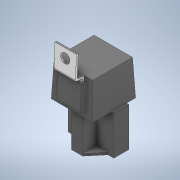
# Autodesk Inventor part: gooacc_30A_spdt
Saved by Autodesk Inventor 2020.2 (Build 242310000, 310)
## iProperties
Created: 2020-04-10
Part Number: gooacc_30A_spdt
Material: PC/ABS Plastic
Document SubType Name: Modeling
Designer: agmlego
Mass: 12.6544 g
Surface Area: 87.4119 cm^2
Volume: 35.4195 cm^3
Density: 0.357273 g/cm^3
Appearance: Smooth - Black
Author: agmlego
Autodesk Inventor part; units mm, degrees
ref_plane "YZ Plane" through (0, 0, 0) normal (1, 0, 0) x (0, 1, 0)
ref_plane "XZ Plane" through (0, 0, 0) normal (0, 1, 0) x (-1, 0, 0)
ref_plane "XY Plane" through (0, 0, 0) normal (0, 0, 1) x (1, 0, 0)
sketch "Sketch1" plane through (0, 0, 0) normal (0, 1, 0) x (-1, 0, 0)
  line L0 (0, 0) -> (27.2, 0)
  line L1 (27.2, 0) -> (27.2, -28.2)
  line L2 (27.2, -28.2) -> (0, -28.2)
  line L3 (0, -28.2) -> (0, 0)
  dimension "d0" = 27.2
  dimension "d1" = 28.2
  constraints: 8 end point, 2 parallel, 1 horizontal, 1 perpendicular
  measures "d0" distance of L0.start L0.end
  measures "d1" distance of L2.end L0.start
extrude "Extrusion1" add sketch "Sketch1" along normal blind 24.9
draft "FaceDraft1" angle 2.5 pull direction (0, 1, 0) faces at (-18.1333, 8.3, 0) (0, 8.3, -9.4) (-9.0667, 8.3, -28.2) (-27.2, 8.3, -18.8) fixed edges at (-13.6, 24.9, 0) (0, 24.9, -14.1) (-13.6, 24.9, -28.2) (-27.2, 24.9, -14.1)
sketch "Sketch2" plane through (-28.2872, 0, 1.0872) normal (0, 0.0436194, 0.9990482) x (1, 0, 0)
  line L0 (4.7872, 21.0237) -> (24.5872, 21.0237)
  line L1 (24.5872, 21.0237) -> (24.5872, 4.0237)
  line L2 (24.5872, 4.0237) -> (4.7872, 4.0237)
  line L3 (4.7872, 4.0237) -> (4.7872, 21.0237)
  line L4 (1.0872, 24.9237) -> (28.2872, 24.9237) construction
  line L5 (14.6872, 24.9237) -> (14.6872, 0) construction
  line L6 (0, 0) -> (29.3743, 0) construction
  point P0 (28.2872, 0.0474)
  point P1 (14.6872, 21.0237)
  dimension "d5" = 19.8
  dimension "d6" = 17
  dimension "d7" = 3.9
  constraints: 10 end point, 3 midpoint, 2 parallel, 1 horizontal, 1 perpendicular, 1 point on line
  measures "d5" distance of L1.end L2.end
  measures "d6" distance of L2.end L0.start
  measures "d7" distance between parallel lines of L4 L0
extrude "Extrusion2" add sketch "Sketch2" along normal blind 2.5
chamfer "Chamfer1" distance 1.75 distance2 2.5 1 edges at (-23.5, 12.6209, 3.0385) measured on face at (-23, 12.6209, 3.0385)
chamfer "Chamfer2" distance 1.75 distance2 2.5 1 edges at (-3.7, 12.6209, 3.0385) measured on face at (-4.2, 12.6209, 3.0385)
sketch "Sketch3" plane through (-23.5, 21.0037, 0.1701) normal (0, 0.9990482, -0.0436194) x (1, 0, 0)
  line L0 (-3.7, 0) -> (23.5, 0) projected
  line L1 (2.3, 0) -> (17.5, 0)
  line L2 (17.5, 0) -> (17.5, -1.2)
  line L3 (17.5, -1.2) -> (2.3, -1.2)
  line L4 (2.3, -1.2) -> (2.3, 0)
  line L5 (9.9, -1.2) -> (9.9, -2.5) construction
  line L6 (1.75, -2.5) -> (18.05, -2.5) construction
  point P0 (23.5, 1.0861)
  point P1 (17.5, 0)
  dimension "d16" = 1.2
  dimension "d17" = 15.2
  constraints: 10 end point, 2 midpoint, 2 parallel, 2 perpendicular, 1 horizontal, 1 point on line
  measures "d16" distance of L3.end L1.start
  measures "d17" distance of L2.end L3.end
extrude "Extrusion3" add sketch "Sketch3" along normal up to surface surface through (-13.6, 24.9, -14.1) normal (0, 1, 0)
sketch "Sketch5" plane through (-21.2, 21.0561, 1.369) normal (0, 0.0436194, 0.9990482) x (1, 0, 0)
  line L0 (15.2, 3.8476) -> (0, 3.8476) projected
  line L1 (15.2, 0) -> (15.2, 3.8476) projected
  line L2 (0, 3.8476) -> (15.2, 3.8476)
  line L3 (15.2, 3.8476) -> (15.2, 2.6476)
  line L4 (15.2, 2.6476) -> (0, 2.6476)
  line L5 (0, 2.6476) -> (0, 3.8476)
  point P0 (21.2, -20.9763)
  dimension "d20" = 1.2
  constraints: 8 end point, 2 parallel, 1 horizontal, 1 perpendicular, 1 point on line
  measures "d20" distance of L4.end L0.end
extrude "Extrusion4" add sketch "Sketch5" along normal blind 5
sketch "Sketch6" plane through (-21.2, 24.9, 1.2011) normal (0, 0.9990482, -0.0436194) x (1, 0, 0)
  line L0 (0, 0) -> (0, -5) projected
  line L1 (0, -3.8) -> (15.2, -3.8)
  line L2 (15.2, -3.8) -> (15.2, -5)
  line L3 (15.2, -5) -> (0, -5)
  line L4 (0, -5) -> (0, -3.8)
  point P0 (21.2, 2.2861)
  dimension "d23" = 1.2
  constraints: 8 end point, 2 parallel, 1 horizontal, 1 perpendicular, 1 point on line
  measures "d23" distance between parallel lines of L3 L1
extrude "Extrusion5" add sketch "Sketch6" along normal blind 15.4
sketch "Sketch7" plane through (-21.2, 21.2742, 6.3642) normal (0, 0.0436194, 0.9990482) x (1, 0, 0)
  circle A0 centre (7.6, 13.2176) radius 3.22 construction
  line L0 (15.2, 19.2476) -> (0, 19.2476) construction
  line L1 (7.6, 19.2476) -> (7.6, 2.6476) construction
  line L2 (0, 2.6476) -> (15.2, 2.6476) construction
  point P0 (21.2, -20.9763)
  dimension "d26" = 6.44
  dimension "d27" = 6.03
  constraints: 2 end point, 2 midpoint, 1 centre point, 1 coincident, 1 point on line
  measures "d26" diameter of A0
  measures "d27" distance from line of L0 A0.centre
hole "Hole1" at (-13.6, 34.4792, 5.7877) direction (0, -0.0436194, -0.9990482) diameter 6.44 end through all start extended yes
fillet "Fillet1" radius 1.2 3 edges at (-13.6, 23.9192, 6.2487) (-13.6, 23.7011, 1.2535) (-13.6, 25.0658, 4.9975)
sketch "Sketch8" plane through (0, 0, 0) normal (0, -1, 0) x (1, 0, 0)
  line L0 (2.75, -22.7872) -> (-8.45, -22.7872)
  line L1 (-8.45, -22.7872) -> (-8.45, -29.2872)
  line L2 (-8.45, -29.2872) -> (-18.75, -29.2872)
  line L3 (-18.75, -29.2872) -> (-18.75, -22.7872)
  line L4 (-18.75, -22.7872) -> (-29.65, -22.7872)
  line L5 (-29.65, -22.7872) -> (-29.65, -12.1872)
  line L6 (-29.65, -12.1872) -> (-17.55, -12.1872)
  line L7 (-17.55, -12.1872) -> (-17.55, -2.4872)
  line L8 (-17.55, -2.4872) -> (-9.55, -2.4872)
  line L9 (-9.55, -2.4872) -> (-9.55, -12.1872)
  line L10 (-9.55, -12.1872) -> (2.75, -12.1872)
  line L11 (2.75, -12.1872) -> (2.75, -22.7872)
  line L12 (1.0872, -29.2872) -> (-28.2872, -29.2872) construction
  point P0 (0, 0)
  point P1 (-13.6, -29.2872)
  dimension "d36" = 10.3
  dimension "d37" = 6.5
  dimension "d38" = 10.9
  dimension "d39" = 10.6
  dimension "d40" = 12.1
  dimension "d41" = 8
  dimension "d42" = 9.7
  dimension "d43" = 11.2
  dimension "d44" = 12.3
  constraints: 24 end point, 9 perpendicular, 4 point on line, 2 midpoint, 1 horizontal
  measures "d36" distance of L1.end L2.end
  measures "d37" distance of L2.end L3.end
  measures "d38" distance of L3.end L4.end
  measures "d39" distance of L4.end L5.end
  measures "d40" distance of L5.end L6.end
  measures "d41" distance of L7.end L8.end
  measures "d42" distance of L6.end L7.end
  measures "d43" distance of L0.start L0.end
  measures "d44" distance of L9.end L10.end
extrude "Extrusion6" add sketch "Sketch8" along normal blind 27.65
sketch "Sketch9" plane through (0, -27.65, 0) normal (0, -1, 0) x (1, 0, 0)
  line L0 (-9.55, -12.1872) -> (1.0872, -12.1872) projected
  line L1 (-9.55, -12.1872) -> (-1.4, -12.1872)
  line L2 (-1.4, -12.1872) -> (-9.55, -2.4872)
  line L3 (-9.55, -2.4872) -> (-9.55, -12.1872) projected
  line L4 (-9.55, -12.1872) -> (-9.55, -2.4872)
  line L5 (-17.55, -2.4872) -> (-17.55, -12.1872) projected
  line L6 (-17.55, -2.4872) -> (-23.95, -12.1872)
  line L7 (-17.55, -12.1872) -> (-29.65, -12.1872) projected
  line L8 (-23.95, -12.1872) -> (-17.55, -12.1872)
  line L9 (-17.55, -12.1872) -> (-17.55, -2.4872)
  line L10 (2.75, -22.7872) -> (2.75, -12.1872) projected
  point P0 (0, 0)
  dimension "d47" = 5.7
  dimension "d48" = 4.15
  constraints: 12 end point, 2 perpendicular, 2 point on line, 1 collinear
  measures "d47" distance of L7.end L6.end
  measures "d48" distance from line of L1.end L10
extrude "Extrusion7" add sketch "Sketch9" against normal blind 1.6
sketch "Sketch10" plane through (0, -27.65, 0) normal (0, -1, 0) x (1, 0, 0)
  line L0 (-18.75, -29.2872) -> (-8.45, -29.2872) construction
  line L1 (-13.6, -29.2872) -> (-13.55, -2.4872) construction
  line L2 (-17.55, -2.4872) -> (-9.55, -2.4872) construction
  line L3 (2.75, -22.7872) -> (2.75, -12.1872) construction
  line L4 (2.75, -17.4872) -> (-29.65, -17.4872) construction
  line L5 (-29.65, -12.1872) -> (-29.65, -22.7872) construction
  line L6 (-8.45, -22.7872) -> (2.75, -22.7872) construction
  line L7 (-2.85, -22.7872) -> (-2.85, -17.4872) construction
  line L8 (-13.5939, -26.0372) -> (-8.45, -26.0372) construction
  line L9 (-8.45, -29.2872) -> (-8.45, -22.7872) construction
  line L10 (-24.2, -17.4872) -> (-24.2, -22.7872) construction
  line L11 (-29.65, -22.7872) -> (-18.75, -22.7872) construction
  line L12 (-13.5591, -7.3506) -> (-20.75, -7.3372) construction
  line L13 (-23.95, -12.1872) -> (-17.55, -2.4872) construction
  point P0 (0, 0)
  point P1 (-13.578, -17.4872)
  constraints: 12 end point, 8 midpoint, 6 point on line, 4 perpendicular
body "Solid1"
